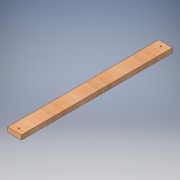
# Autodesk Inventor part: CarrierBracket
Saved by Autodesk Inventor 2016 (Build 200138000, 138)
## iProperties
Created: 2016-01-18
Part Number: CarrierBracket
Material: Wood (Birch)
Document SubType Name: Modeling
Designer: yash
Density: 0.55 g/cm^3
Appearance: Birch - Natural Polished
Author: yash
Autodesk Inventor part; units mm, degrees
ref_plane "YZ Plane" through (0, 0, 0) normal (1, 0, 0) x (0, 1, 0)
ref_plane "XZ Plane" through (0, 0, 0) normal (0, 1, 0) x (-1, 0, 0)
ref_plane "XY Plane" through (0, 0, 0) normal (0, 0, 1) x (1, 0, 0)
sketch "Sketch1" plane through (0, 0, 0) normal (0, 1, 0) x (-1, 0, 0)
  line L0 (0, 0) -> (76.2, 0)
  line L1 (76.2, 0) -> (76.2, -838.2)
  line L2 (76.2, -838.2) -> (0, -838.2)
  line L3 (0, -838.2) -> (0, 0)
  dimension "d0" = 76.2
  dimension "d1" = 838.2
  constraints: 8 end point, 2 parallel, 1 horizontal, 1 perpendicular
  measures "d0" distance of L1.end L2.end
  measures "d1" distance of L0.end L1.end
extrude "Extrusion1" add sketch "Sketch1" along normal blind 25.4
sketch "Sketch2" plane through (0, 25.4, 0) normal (0, 1, 0) x (1, 0, 0)
  line L0 (-76.2, 0) -> (0, 0) projected
  line L1 (-76.2, 838.2) -> (-76.2, 0) projected
  point P0 (-38.1, 25.4)
  point P1 (-38.1, 812.8)
  point P2 (-38.1, 419.1)
  point P3 (-38.1, 0)
  point P4 (-76.2, 419.1)
  dimension "d4" = 787.4
  dimension "d5" = 393.7
  constraints: 3 vertical alignment, 2 midpoint, 1 horizontal alignment
  measures "d4" distance of point (-38.1, 25.4) point (-38.1, 812.8)
  measures "d5" distance of point (-38.1, 25.4) point (-38.1, 419.1)
hole "Hole1" at (-38.1, 25.4, -812.8) at (-38.1, 25.4, -25.4) direction (0, -1, 0) diameter 6.35 end through all
equation "\"d5\" = 0.5 * d4"
body "Solid1"
